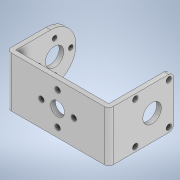
# Autodesk Inventor part: Part1
Saved by Autodesk Inventor 2021 (Build 250183000, 183)
## iProperties
Created: 2021-10-22
Part Number: Part1
Material: Generic
Document SubType Name: Modeling
Designer: Asus
Density: 1 g/cm^3
Appearance: Default
Author: Asus
Autodesk Inventor part; units mm, degrees
ref_plane "YZ Plane" through (0, 0, 0) normal (1, 0, 0) x (0, 1, 0)
ref_plane "XZ Plane" through (0, 0, 0) normal (0, 1, 0) x (-1, 0, 0)
ref_plane "XY Plane" through (0, 0, 0) normal (0, 0, 1) x (1, 0, 0)
sketch "Sketch1" plane through (0, 0, 0) normal (0, 0, 1) x (1, 0, 0)
  line L0 (0, 0) -> (44.2, 0)
  line L1 (44.2, 0) -> (44.2, 21.8)
  line L2 (44.2, 21.8) -> (0, 21.8)
  line L3 (0, 21.8) -> (0, 0)
  dimension "d0" = 21.8
  dimension "d1" = 44.2
  constraints: 8 end point, 2 parallel, 1 horizontal, 1 perpendicular
  measures "d0" distance of L1.end L0.end
  measures "d1" distance of L1.end L2.end
extrude "Extrusion1" add sketch "Sketch1" along normal blind 2
sketch "Sketch2" plane through (0, 0, 0) normal (0, 0, -1) x (-1, 0, 0)
  line L0 (0, 21.8) -> (-2, 21.8)
  line L1 (-2, 21.8) -> (-2, 0)
  line L2 (-2, 0) -> (0, 0)
  line L3 (0, 0) -> (0, 21.8)
  line L4 (-44.2, 0) -> (-44.2, 21.8) projected
  line L5 (0, 0) -> (-44.2, 0) projected
  line L6 (-44.2, 21.8) -> (-42.2, 21.8)
  line L7 (-42.2, 21.8) -> (-42.2, 0)
  line L8 (-42.2, 0) -> (-44.2, 0)
  line L9 (-44.2, 0) -> (-44.2, 21.8)
  dimension "d4" = 2
  dimension "d5" = 2
  dimension "d93" = 21.8
  constraints: 16 end point, 4 parallel, 2 horizontal, 2 perpendicular, 1 point on line
  measures "d4" distance of L2.end L1.end
  measures "d5" distance of L7.end L8.end
  measures "d93" distance of L0.end L1.end
extrude "Extrusion2" add sketch "Sketch2" along normal blind 26
fillet "Fillet1" radius 10.9 2 edges at (1, 21.8, -26) (1, 0, -26)
fillet "Fillet2" radius 2 2 edges at (43.2, 21.8, -26) (43.2, 0, -26)
sketch "Sketch3" plane through (0, 0, 2) normal (-1, 0, 0) x (0, 0, 1)
  line L0 (-28, 19.8) -> (-28, 2) projected
  circle A0 centre (-18.75, 10.9) radius 7
  circle A1 centre (-25.75, 10.9) radius 1
  circle A2 centre (-18.75, 3.9) radius 1
  circle A3 centre (-11.75, 10.9) radius 1
  circle A4 centre (-18.75, 17.9) radius 1
  point P0 (-2, 0)
  dimension "d11" = 14
  dimension "d12" = 2
  dimension "d15" = 360
  constraints: 4 centre point, 1 coincident, 1 horizontal alignment, 11 other
  measures "d12" diameter of A1
hole "Hole1" at (0, 17.9, -16.75) at (0, 10.9, -23.75) at (0, 3.9, -16.75) at (0, 10.9, -9.75) direction (1, 0, 0) diameter 2 depth 2
thread "Thread1" size "M2x0.4" class "6H" standard "ANSI Metric M Profile" length 2
thread "Thread2" size "M2x0.4" class "6H" standard "ANSI Metric M Profile" length 2
thread "Thread3" size "M2x0.4" class "6H" standard "ANSI Metric M Profile" length 2
thread "Thread4" size "M2x0.4" class "6H" standard "ANSI Metric M Profile" length 2
sketch "Sketch4" plane through (44.2, 0, 2) normal (1, 0, 0) x (0, 0, -1)
  line L0 (26, 21.8) -> (0, 21.8) projected
  arc A0 (28, 19.8) -> (26, 21.8) centre (26, 19.8) ccw projected
  circle A1 centre (11.5, 19.8) radius 1
  circle A2 centre (26, 19.8) radius 1
  line L1 (26, 0) -> (26, 2)
  circle A3 centre (26, 2) radius 1
  circle A4 centre (11.5, 2) radius 1
  point P0 (2, 0)
  dimension "d34" = 2
  dimension "d35" = 2
  dimension "d36" = 2
  dimension "d37" = 2
  dimension "d38" = 2
  constraints: 4 centre point, 2 coincident, 2 end point, 1 vertical
  measures "d34" diameter of A1
  measures "d35" diameter of A2
  measures "d36" distance of L1.start L1.end
  measures "d37" diameter of A3
  measures "d38" diameter of A4
hole "Hole2" at (44.2, 19.8, -9.5) at (44.2, 19.8, -24) at (44.2, 2, -24) at (44.2, 2, -9.5) direction (-1, 0, 0) diameter 2 depth 2
thread "Thread5" size "M2x0.4" class "6H" standard "ANSI Metric M Profile" length 2
thread "Thread6" size "M2x0.4" class "6H" standard "ANSI Metric M Profile" length 2
thread "Thread7" size "M2x0.4" class "6H" standard "ANSI Metric M Profile" length 2
thread "Thread8" size "M2x0.4" class "6H" standard "ANSI Metric M Profile" length 2
fillet "Fillet3" radius 2 2 edges at (0, 10.9, 2) (44.2, 10.9, 2)
sketch "Sketch5" plane through (0, 21.8, -15.1) normal (-1, 0, 0) x (0, 0, 1)
  circle A0 centre (-1.65, -3.9) radius 1 projected
  circle A1 centre (-1.65, -17.9) radius 1 projected
  line L0 (-1.65, -3.9) -> (-1.65, -17.9)
  circle A2 centre (-1.65, -10.9) radius 4
  point P0 (15.1, -21.8)
  dimension "d55" = 8
  constraints: 2 end point, 1 centre point, 1 midpoint, 1 vertical
  measures "d55" diameter of A2
hole "Hole3" at (0, 10.9, -16.75) direction (1, 0, 0) diameter 8 depth 44.75
sketch "Sketch6" plane through (0, 0, 2) normal (0, 0, 1) x (1, 0, 0)
  line L0 (2, 0) -> (42.2, 0) projected
  line L1 (22.1, 0) -> (22.1, 21.8)
  line L2 (42.2, 21.8) -> (2, 21.8) projected
  line L3 (44.4097, 10.9) -> (-11.7207, 10.9)
  circle A0 centre (22.1, 10.9) radius 3
  circle A1 centre (22.1, 10.9) radius 7
  circle A2 centre (22.1, 3.9) radius 1
  circle A3 centre (29.1, 10.9) radius 1
  circle A4 centre (22.1, 17.9) radius 1
  circle A5 centre (15.1, 10.9) radius 1
  point P0 (0, 0)
  dimension "d64" = 14
  dimension "d63" = 6
  dimension "d65" = 2
  dimension "d68" = 360
  constraints: 5 centre point, 4 end point, 3 midpoint, 2 point on line, 1 coincident, 1 horizontal, 1 vertical alignment, 11 other
  measures "d63" diameter of A0
  measures "d65" diameter of A2
hole "Hole4" at (22.1, 3.9, 2) at (29.1, 10.9, 2) at (22.1, 17.9, 2) at (15.1, 10.9, 2) direction (0, 0, -1) diameter 2 depth 2
sketch "Sketch7" plane through (0, 0, 2) normal (0, 0, 1) x (1, 0, 0)
  circle A0 centre (22.1, 3.9) radius 1 projected
  circle A1 centre (22.1, 17.9) radius 1 projected
  line L0 (22.1, 3.9) -> (22.1, 17.9)
  circle A2 centre (22.1, 10.9) radius 3
  point P0 (0, 0)
  dimension "d77" = 6
  constraints: 2 end point, 1 centre point, 1 midpoint, 1 vertical
  measures "d77" diameter of A2
hole "Hole5" at (22.1, 10.9, 2) direction (0, 0, -1) diameter 6 depth 2
thread "Thread9" size "M2x0.4" class "6H" standard "ANSI Metric M Profile" length 2
thread "Thread10" size "M2x0.4" class "6H" standard "ANSI Metric M Profile" length 2
thread "Thread11" size "M2x0.4" class "6H" standard "ANSI Metric M Profile" length 2
thread "Thread12" size "M2x0.4" class "6H" standard "ANSI Metric M Profile" length 2
chamfer "Chamfer1" distance 0.2 angle 45 12 edges at (44.2, 2, -8.5) (44.2, 19.8, -8.5) (44.2, 2, -23) (44.2, 19.8, -23) (22.1, 4.9, 2) (15.1, 11.9, 2) (29.1, 11.9, 2) (22.1, 18.9, 2) (0, 10.9, -10.75) (0, 17.9, -17.75) (0, 3.9, -17.75) (0, 10.9, -24.75)
body "Solid1"
